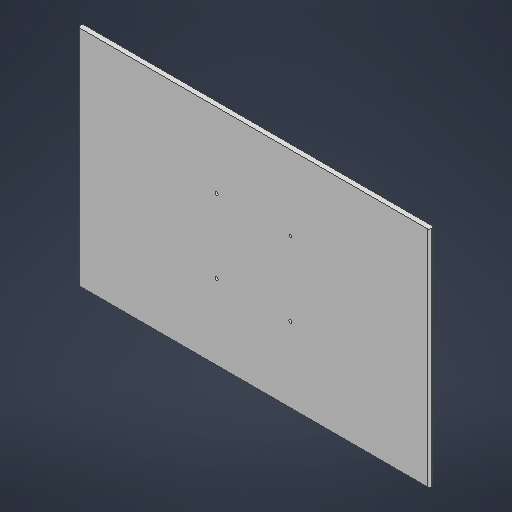
# Autodesk Inventor part: Monitor
Saved by Autodesk Inventor 2025.1 (Build 291241000, 241)
## iProperties
Created: 2025-02-19
Part Number: Monitor
Material: Generic
Document SubType Name: Modeling
Designer: jerem
Density: 1 g/cm^3
Appearance: Default
Author: jerem
Autodesk Inventor part; units mm, degrees
ref_plane "YZ Plane" through (0, 0, 0) normal (1, 0, 0) x (0, 1, 0)
ref_plane "XZ Plane" through (0, 0, 0) normal (0, 1, 0) x (-1, 0, 0)
ref_plane "XY Plane" through (0, 0, 0) normal (0, 0, 1) x (1, 0, 0)
sketch "Sketch1" plane through (0, 0, 0) normal (0, 0, 1) x (1, 0, 0)
  line L0 (178.5, -113.5) -> (-178.5, -113.5)
  line L1 (-178.5, -113.5) -> (-178.5, 113.5)
  line L2 (-178.5, 113.5) -> (178.5, 113.5)
  line L3 (178.5, 113.5) -> (178.5, -113.5)
  line L4 (178.5, -113.5) -> (-178.5, 113.5) construction
  line L5 (-178.5, -113.5) -> (178.5, 113.5) construction
  point P0 (0, 0)
  dimension "d0" = 357
  dimension "d1" = 227
  constraints: 12 end point, 2 midpoint, 2 parallel, 1 horizontal, 1 perpendicular
  measures "d0" distance of L1.end L2.end
  measures "d1" distance of L0.end L1.end
extrude "Extrusion1" add sketch "Sketch1" along normal blind 5
sketch "Sketch2" plane through (0, 0, 5) normal (0, 0, 1) x (1, 0, 0)
  line L0 (37.5, -37.5) -> (-37.5, -37.5) construction
  line L1 (-37.5, -37.5) -> (-37.5, 37.5) construction
  line L2 (-37.5, 37.5) -> (37.5, 37.5) construction
  line L3 (37.5, 37.5) -> (37.5, -37.5) construction
  line L4 (37.5, -37.5) -> (-37.5, 37.5) construction
  line L5 (-37.5, -37.5) -> (37.5, 37.5) construction
  point P0 (0, 0)
  dimension "d4" = 75
  dimension "d5" = 75
  constraints: 12 end point, 4 coincident, 2 midpoint, 2 parallel, 1 horizontal, 1 perpendicular
  measures "d4" distance of L1.end L2.end
  measures "d5" distance of L0.end L1.end
hole "Hole1" at (-37.5, 37.5, 5) at (37.5, 37.5, 5) at (37.5, -37.5, 5) at (-37.5, -37.5, 5) direction (0, 0, -1) diameter 3 depth 3
fillet "Fillet1" radius 2 4 edges at (-178.5, 0, 0) (-178.5, 0, 5) (178.5, 0, 5) (178.5, 0, 0)
sketch "Sketch3" plane through (0, 0, 0) normal (0, 0, -1) x (-1, 0, 0)
  line L0 (168.1886, -102.5002) -> (-168.1886, -102.5002)
  line L1 (-168.1886, -102.5002) -> (-168.1886, 102.5002)
  line L2 (-168.1886, 102.5002) -> (168.1886, 102.5002)
  line L3 (168.1886, 102.5002) -> (168.1886, -102.5002)
  line L4 (168.1886, -102.5002) -> (-168.1886, 102.5002) construction
  line L5 (-168.1886, -102.5002) -> (168.1886, 102.5002) construction
  point P0 (0, 0)
  constraints: 12 end point, 2 midpoint, 2 parallel, 1 horizontal, 1 perpendicular
extrude "Extrusion2" cut sketch "Sketch3" against normal blind 1
body "Solid1"
